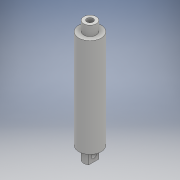
# Autodesk Inventor part: cylinder
Saved by Autodesk Inventor 2017 (Build 210142000, 142)
## iProperties
Created: 2018-01-02
Part Number: cylinder
Material: Generic
Document SubType Name: Modeling
Designer: RLanting
Density: 1 g/cm^3
Appearance: Default
Author: RLanting
Autodesk Inventor part; units mm, degrees
ref_plane "YZ Plane" through (0, 0, 0) normal (1, 0, 0) x (0, 1, 0)
ref_plane "XZ Plane" through (0, 0, 0) normal (0, 1, 0) x (-1, 0, 0)
ref_plane "XY Plane" through (0, 0, 0) normal (0, 0, 1) x (1, 0, 0)
sketch "Sketch1" plane through (0, 0, 0) normal (0, 0, 1) x (1, 0, 0)
  circle A0 centre (0, 0) radius 14.25
  dimension "d0" = 28.5
  constraints: 1 centre point, 1 coincident
  measures "d0" diameter of A0
extrude "Extrusion1" add sketch "Sketch1" along normal blind 125
sketch "Sketch2" plane through (0, 0, 125) normal (0, 0, 1) x (1, 0, 0)
  circle A0 centre (0, 0) radius 7.9375
  dimension "d3" = 15.875
  constraints: 1 centre point, 1 coincident
  measures "d3" diameter of A0
extrude "Extrusion2" add sketch "Sketch2" along normal blind 12.5
sketch "Sketch3" plane through (0, 0, 137.5) normal (0, 0, 1) x (1, 0, 0)
  circle A0 centre (0, 0) radius 4
  dimension "d6" = 8
  constraints: 1 centre point, 1 coincident
  measures "d6" diameter of A0
extrude "Extrusion3" cut sketch "Sketch3" against normal blind 50.8
sketch "Sketch4" plane through (0, 0, 0) normal (0, 0, -1) x (-1, 0, 0)
  circle A0 centre (0, 0) radius 7.9375
  dimension "d9" = 15.875
  constraints: 1 centre point, 1 coincident
  measures "d9" diameter of A0
extrude "Extrusion4" add sketch "Sketch4" along normal blind 16
sketch "Sketch5" plane through (0, 0, -16) normal (0, 0, -1) x (-1, 0, 0)
  line L0 (-4.75, -7.9375) -> (4.75, -7.9375)
  line L1 (4.75, -7.9375) -> (4.75, 7.9375)
  line L2 (4.75, 7.9375) -> (-4.75, 7.9375)
  line L3 (-4.75, 7.9375) -> (-4.75, -7.9375)
  line L4 (-4.75, -7.9375) -> (4.75, 7.9375) construction
  line L5 (4.75, -7.9375) -> (-4.75, 7.9375) construction
  circle A0 centre (0, 0) radius 7.9375 construction
  circle A1 centre (0, 0) radius 7.9375 projected
  arc A2 (-4.8155, 6.3099) -> (-4.8155, -6.3099) centre (0, 0) ccw
  arc A3 (4.7611, -6.351) -> (4.7611, 6.351) centre (0, 0) ccw
  line L6 (-4.8155, 6.3099) -> (-4.8155, -6.3099)
  line L7 (4.7611, 6.351) -> (4.7611, -6.351)
  dimension "d12" = 9.5
  constraints: 16 end point, 8 point on circle, 4 parallel, 2 centre point, 2 coincident, 2 midpoint, 1 horizontal, 1 perpendicular, 1 tangent
  measures "d12" distance between parallel lines of L1 L3
extrude "Extrusion5" cut sketch "Sketch5" against normal up to surface (16 mm away) contours A1 L6 | L7 A1
sketch "Sketch6" plane through (4.8155, -6.3099, -16) normal (1, 0, 0) x (0, 0, -1)
  line L0 (0, -0.0411) -> (0, 12.6609) construction
  line L1 (0, 6.3099) -> (-7, 6.3099) construction
  circle A0 centre (-7, 6.3099) radius 3.2
  point P0 (-16, 6.3099)
  dimension "d15" = 6.4
  dimension "d16" = 7
  constraints: 2 end point, 1 centre point, 1 coincident, 1 horizontal, 1 midpoint
  measures "d15" diameter of A0
  measures "d16" distance of L1.start L1.end
extrude "Extrusion6" cut sketch "Sketch6" against normal through all
body "Solid1"
